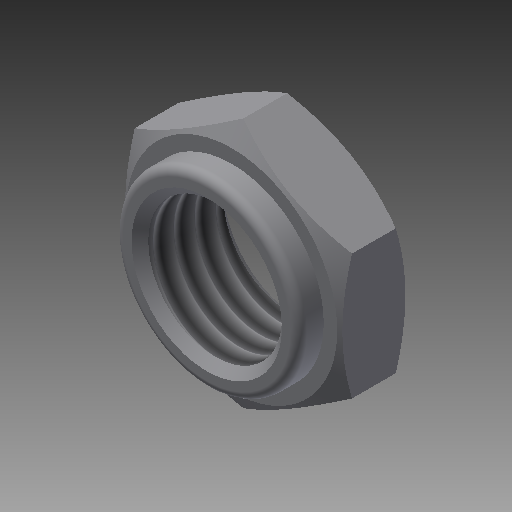
# Autodesk Inventor part: Dado 13
Saved by Autodesk Inventor 2019 (Build 230136000, 136)
## iProperties
Created: 2011-09-22
Part Number: Dado 13
Document SubType Name: Modeling
Designer: Stefano
Density: 1 g/cm^3
Material: 一般
Appearance: 既定
Author: Stefano
Autodesk Inventor part; units mm, degrees
ref_plane "YZ Plane" through (0, 0, 0) normal (1, 0, 0) x (0, 1, 0)
ref_plane "XZ Plane" through (0, 0, 0) normal (0, 1, 0) x (-1, 0, 0)
ref_plane "XY Plane" through (0, 0, 0) normal (0, 0, 1) x (1, 0, 0)
sketch "Schizzo1" plane through (0, 0, 0) normal (0, 0, 1) x (1, 0, 0)
  line L0 (0, 7.5056) -> (6.5, 3.7528)
  line L1 (6.5, 3.7528) -> (6.5, -3.7528)
  line L2 (6.5, -3.7528) -> (0, -7.5056)
  line L3 (0, -7.5056) -> (-6.5, -3.7528)
  line L4 (-6.5, -3.7528) -> (-6.5, 3.7528)
  line L5 (-6.5, 3.7528) -> (0, 7.5056)
  point P0 (0, 0)
  point P1 (0, 0)
  dimension "d0" = 13
  constraints: 12 end point, 1 coincident, 13 other
  measures "d0" distance between parallel lines of L1 L4
extrude "Estrusione1" add sketch "Schizzo1" along normal blind 4
sketch "Schizzo2" plane through (0, 0, 4) normal (0, 0, 1) x (1, 0, 0)
  circle A0 centre (0, 0) radius 5.5
  dimension "d5" = 11
  constraints: 1 centre point, 1 coincident
  measures "d5" diameter of A0
extrude "Estrusione2" add sketch "Schizzo2" along normal blind 1.5
sketch "Schizzo3" plane through (0, 0, 0) normal (1, 0, 0) x (0, 1, 0)
  line L0 (7.5056, 4) -> (3.7528, 4) projected
  line L1 (3.7528, 0) -> (3.7528, 4) projected
  line L2 (7.5056, 0) -> (3.7528, 0) projected
  line L3 (7.5056, 0) -> (7.5056, 4) projected
  line L4 (6.3093, 0) -> (7.5056, 0.6907)
  line L5 (0, -1) -> (0, 6) projected
  line L6 (6.3093, 4) -> (7.5056, 4)
  line L7 (6.3093, 4) -> (7.5056, 3.3093)
  point P0 (0, 0)
  dimension "d6" = 30
  dimension "d23" = 30
  constraints: 6 end point, 3 point on line, 1 collinear
  measures "d6" angle of L4 L2
  measures "d23" angle of L0 L7
ref_plane "Piano di lavoro1" through (0, 0, 2) normal (0, 0, -1) x (-1, 0, 0)
sketch "Schizzo4" plane through (0, 0, 5.5) normal (0, 0, 1) x (1, 0, 0)
  circle A0 centre (0, 0) radius 5.5 projected
hole "Foro1" at (0, 0, 5.5) direction (0, 0, -1) diameter 8 end through all
thread "Filettatura1" size "M9x1.25" class "6H" standard "ANSI Metric M Profile" full length
chamfer "Smusso1" distance 0.5 angle 45 2 edges at (0, 4, 5.5) (0, 4, 0)
revolve "Rivoluzione2" cut sketch "Schizzo3" angle 360 about axis through (0, 0, -10) along (0, 0, 1) contours L3 L7 L0 | L3 L2 L4
fillet "Raccordo1" radius 0.5 1 edges at (-5.5, 0, 5.5)
